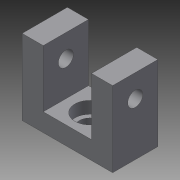
# Autodesk Inventor part: Arm_Pulley_Connector
Saved by Autodesk Inventor 2015 (Build 190159000, 159)
## iProperties
Created: 2017-03-09
Part Number: Arm_Pulley_Connector
Material: Generic
Document SubType Name: Modeling
Designer: Guy
Density: 1 g/cm^3
Appearance: Default
Author: Guy
Autodesk Inventor part; units mm, degrees
ref_plane "YZ Plane" through (0, 0, 0) normal (1, 0, 0) x (0, 1, 0)
ref_plane "XZ Plane" through (0, 0, 0) normal (0, 1, 0) x (-1, 0, 0)
ref_plane "XY Plane" through (0, 0, 0) normal (0, 0, 1) x (1, 0, 0)
sketch "Sketch1" plane through (0, 0, 0) normal (0, 0, 1) x (1, 0, 0)
  line L0 (0, 0) -> (30, 0)
  line L1 (30, 0) -> (30, 15)
  line L2 (30, 15) -> (0, 15)
  line L3 (0, 15) -> (0, 0)
  dimension "d0" = 30
  dimension "d1" = 15
  constraints: 8 end point, 2 parallel, 1 horizontal, 1 perpendicular
  measures "d0" distance of L2.end L1.end
  measures "d1" distance of L2.end L0.start
extrude "Extrusion1" add sketch "Sketch1" along normal blind 25
sketch "Sketch2" plane through (0, 15, 0) normal (0, 1, 0) x (1, 0, 0)
  line L0 (30, 0) -> (0, 0) projected
  line L1 (0, 0) -> (0, -25) projected
  line L2 (30, -25) -> (0, -25) projected
  line L3 (30, 0) -> (30, -25) projected
  line L4 (7, -25) -> (23, -25)
  line L5 (23, -25) -> (23, -6)
  line L6 (23, -6) -> (7, -6)
  line L7 (7, -6) -> (7, -25)
  point P0 (0, 0)
  dimension "d5" = 16
  dimension "d27" = 7
  dimension "d28" = 6
  constraints: 8 end point, 2 parallel, 1 horizontal, 1 perpendicular, 1 point on line
  measures "d5" distance between parallel lines of L5 L7
  measures "d27" distance between parallel lines of L1 L7
  measures "d28" distance between parallel lines of L0 L6
extrude "Extrusion2" cut sketch "Sketch2" against normal up to next contours L2 L7 L6 L5
sketch "Sketch3" plane through (30, 0, 0) normal (1, 0, 0) x (0, 0, -1)
  circle A0 centre (-17.5, 7.5) radius 2.5
  line L0 (-25, 0) -> (-25, 15) projected
  line L1 (0, 15) -> (-25, 15) projected
  point P0 (0, 0)
  dimension "d10" = 5
  dimension "d11" = 7.5
  dimension "d12" = 7.5
  constraints: 1 centre point
  measures "d10" diameter of A0
  measures "d11" distance from line of L0 A0.centre
  measures "d12" distance from line of L1 A0.centre
extrude "Extrusion3" cut sketch "Sketch3" against normal through all
sketch "Sketch6" plane through (7, 15, 6) normal (0, 0, 1) x (1, 0, 0)
  circle A0 centre (8, -7.5) radius 5
  line L0 (0, 0) -> (16, 0) projected
  line L1 (16, 0) -> (16, -15) projected
  point P0 (-7, -15)
  dimension "d29" = 10
  dimension "d30" = 7.5
  dimension "d31" = 8
  constraints: 1 centre point
  measures "d29" diameter of A0
  measures "d30" distance from line of A0.centre L0
  measures "d31" distance from line of L1 A0.centre
extrude "Extrusion6" cut sketch "Sketch6" against normal blind 4
sketch "Sketch7" plane through (15, 7.5, 2) normal (0, 0, 1) x (1, 0, 0)
  circle A0 centre (0, 0) radius 3.5
  point P0 (-15, -7.5)
  dimension "d34" = 7
  constraints: 1 centre point
  measures "d34" diameter of A0
extrude "Extrusion7" cut sketch "Sketch7" against normal up to next
body "Solid1"
